Autodesk Inventor part; units mm, degrees
(part 2 of 6)
sketch "S03_340p2" plane through (0, 0, 0) normal (0, 0, 1) x (1, 0, 0)
  spline S0 degree 4 poles (238.0768, -5.4859) (238.0262, -5.474) (237.779, -5.4146) (237.364, -5.3165) (236.6634, -5.1506) (235.9264, -4.9756) (235.0209, -4.7632) (233.9546, -4.5121) (232.7252, -4.2255) (231.3359, -3.902) (229.7872, -3.5447) (228.0804, -3.1524) (226.2178, -2.7277) (224.2001, -2.2712) (222.0305, -1.7836) (219.7094, -1.2675) (217.2402, -0.7231) (214.625, -0.1526) (211.8658, 0.4439) (208.9653, 1.0631) (205.9266, 1.7045) (202.7523, 2.3663) (199.4449, 3.0472) (196.0087, 3.7454) (192.4456, 4.4591) (188.7604, 5.1862) (184.955, 5.9264) (181.0347, 6.6766) (177.0015, 7.4365) (172.8611, 8.2025) (168.6158, 8.9751) (164.2708, 9.7507) (159.8297, 10.529) (155.2973, 11.3074) (150.6772, 12.0849) (145.9752, 12.8596) (141.1941, 13.6294) (136.34, 14.3935) (131.4172, 15.1492) (126.4302, 15.8959) (121.3842, 16.6311) (116.2838, 17.3537) (111.1345, 18.0622) (105.9413, 18.7549) (100.7087, 19.4294) (95.443, 20.0851) (90.1479, 20.7208) (84.8303, 21.3331) (79.494, 21.9228) (74.1456, 22.4868) (68.7891, 23.0248) (63.4312, 23.5346) (58.0761, 24.0141) (52.7299, 24.4647) (47.3975, 24.8819) (42.08, 25.2672) (36.7914, 25.6169) (31.5078, 25.9337) (26.2453, 26.1996) (21.0236, 26.419) (15.8442, 26.589) (10.716, 26.7093) (5.6442, 26.7813) (0.6348, 26.8019) (-4.3081, 26.7748) (-9.1776, 26.6965) (-13.9701, 26.5701) (-18.6795, 26.3941) (-23.3014, 26.171) (-27.8303, 25.8995) (-32.2623, 25.5822) (-36.5918, 25.2189) (-40.8146, 24.8118) (-44.9265, 24.3608) (-48.9229, 23.8689) (-52.7993, 23.3366) (-56.5528, 22.7661) (-60.1783, 22.1582) (-63.673, 21.5164) (-67.0326, 20.8409) (-70.2544, 20.1338) (-73.3348, 19.3988) (-76.2708, 18.6358) (-79.0595, 17.8478) (-81.6988, 17.0376) (-84.1852, 16.2058) (-86.5171, 15.3554) (-88.6923, 14.4885) (-90.7089, 13.6063) (-92.5646, 12.7109) (-94.2592, 11.8045) (-95.7904, 10.8887) (-97.157, 9.9637) (-98.3599, 9.0328) (-99.3959, 8.0942) (-100.2663, 7.1501) (-100.9698, 6.2002) (-101.5046, 5.2436) (-101.867, 4.2806) (-102.0565, 3.315) (-102.0685, 2.3484) (-101.9089, 1.395) (-101.5753, 0.4697) (-101.0719, -0.4267) (-100.4022, -1.2915) (-99.569, -2.1257) (-98.5748, -2.9295) (-97.4206, -3.7051) (-96.1081, -4.4524) (-94.638, -5.1717) (-93.0118, -5.863) (-91.2313, -6.5259) (-89.2977, -7.1607) (-87.2135, -7.7667) (-84.9804, -8.3444) (-82.6012, -8.8925) (-80.0775, -9.4126) (-77.4128, -9.9023) (-74.609, -10.3636) (-71.6695, -10.7959) (-68.5965, -11.1986) (-65.3939, -11.5716) (-62.0641, -11.9176) (-58.6109, -12.2331) (-55.0375, -12.5221) (-51.3466, -12.7824) (-47.5428, -13.0161) (-43.6291, -13.2239) (-39.6094, -13.4046) (-35.4871, -13.5622) (-31.2664, -13.6937) (-26.9512, -13.8041) (-22.5454, -13.891) (-18.0526, -13.9576) (-13.4782, -14.005) (-8.8246, -14.0327) (-4.0979, -14.0442) (0.6989, -14.0393) (5.5607, -14.0194) (10.4834, -13.9869) (15.4623, -13.9431) (20.4929, -13.8877) (25.5736, -13.8249) (30.6965, -13.752) (35.87, -13.6774) (41.1014, -13.5853) (46.3548, -13.48) (51.6364, -13.3596) (56.934, -13.2271) (62.2443, -13.0833) (67.5615, -12.9292) (72.8799, -12.7653) (78.1948, -12.5938) (83.501, -12.4137) (88.7934, -12.2286) (94.0665, -12.0366) (99.3153, -11.8411) (104.5345, -11.6413) (109.7195, -11.4375) (114.8643, -11.2326) (119.9644, -11.0252) (125.0148, -10.816) (130.0105, -10.6074) (134.9458, -10.3977) (139.8171, -10.189) (144.6184, -9.9809) (149.3454, -9.7738) (153.9932, -9.5683) (158.5579, -9.365) (163.0336, -9.1642) (167.4168, -8.9655) (171.7029, -8.7695) (175.8874, -8.5777) (179.9659, -8.3878) (183.9349, -8.2029) (187.7897, -8.0209) (191.5269, -7.8443) (195.1424, -7.6707) (198.6328, -7.5029) (201.994, -7.3394) (205.2234, -7.1814) (208.3166, -7.0282) (211.2715, -6.8818) (214.0843, -6.7401) (216.7525, -6.6055) (219.2732, -6.4775) (221.6439, -6.3552) (223.8618, -6.2408) (225.9253, -6.1339) (227.8314, -6.0336) (229.5784, -5.9419) (231.1648, -5.8574) (232.5882, -5.7821) (233.848, -5.7143) (234.9418, -5.6556) (235.87, -5.6058) (236.6266, -5.5642) (237.3454, -5.5262) (237.7711, -5.5022) (238.0248, -5.4886) (238.0768, -5.4859) knots 0 0 0 0 0 0.003306 0.005253 0.00752 0.010062 0.01285 0.015861 0.019079 0.022488 0.026078 0.029837 0.033757 0.037828 0.042045 0.046398 0.050884 0.055494 0.060224 0.065069 0.070023 0.075082 0.080241 0.085495 0.090841 0.096274 0.101791 0.107386 0.113057 0.118799 0.124609 0.130484 0.136419 0.142412 0.148458 0.154554 0.160697 0.166884 0.17311 0.179374 0.185671 0.191998 0.198352 0.20473 0.211128 0.217543 0.223972 0.230412 0.23686 0.243312 0.249765 0.256217 0.262663 0.2691 0.275526 0.281941 0.288345 0.294734 0.301105 0.307451 0.313767 0.320049 0.326294 0.332498 0.338659 0.344773 0.350837 0.356848 0.362801 0.368695 0.374525 0.380288 0.38598 0.391599 0.39714 0.4026 0.407976 0.413263 0.418458 0.423557 0.428556 0.433452 0.438241 0.442917 0.447478 0.451919 0.456236 0.460425 0.464482 0.468403 0.472185 0.475825 0.479322 0.482675 0.485889 0.48897 0.49193 0.494788 0.497572 0.50031 0.503032 0.505769 0.508552 0.511409 0.514365 0.517441 0.520647 0.523991 0.527474 0.531098 0.534861 0.538758 0.542789 0.546947 0.551231 0.555634 0.560154 0.564786 0.569527 0.574371 0.579315 0.584356 0.58949 0.594712 0.60002 0.605409 0.610877 0.61642 0.622034 0.627716 0.633463 0.639271 0.645138 0.651061 0.657035 0.663059 0.669128 0.675241 0.681393 0.687582 0.693804 0.700057 0.706341 0.712655 0.718998 0.725365 0.731751 0.738149 0.744556 0.750969 0.757385 0.7638 0.770211 0.776616 0.783011 0.789393 0.795759 0.802106 0.808429 0.814727 0.820996 0.827232 0.833433 0.839595 0.845714 0.851788 0.857813 0.863785 0.869702 0.875558 0.881352 0.887078 0.892735 0.898316 0.90382 0.909242 0.914577 0.919822 0.924972 0.930023 0.93497 0.939808 0.944533 0.949139 0.95362 0.95797 0.962183 0.966252 0.970169 0.973927 0.977515 0.980924 0.984141 0.987151 0.989939 0.99248 0.994747 0.996694 1 1 1 1 1
  circle A0 centre (0, 0) radius 5.15
  line L0 (-36.89, 3.1) -> (-26.69, 3.1)
  line L1 (-26.69, 3.1) -> (-26.69, -1.1)
  line L2 (-26.69, -1.1) -> (-36.89, -1.1)
  line L3 (-36.89, -1.1) -> (-36.89, 3.1)
  line L4 (-36.89, 3.1) -> (-26.69, -1.1) construction
  line L5 (-26.69, 3.1) -> (-36.89, -1.1) construction
  line L6 (-73.14, 4.1) -> (-62.94, 4.1)
  line L7 (-62.94, 4.1) -> (-62.94, -0.1)
  line L8 (-62.94, -0.1) -> (-73.14, -0.1)
  line L9 (-73.14, -0.1) -> (-73.14, 4.1)
  line L10 (-73.14, 4.1) -> (-62.94, -0.1) construction
  line L11 (-62.94, 4.1) -> (-73.14, -0.1) construction
  line L12 (55.1, 4.1) -> (44.9, 4.1)
  line L13 (44.9, 4.1) -> (44.9, -0.1)
  line L14 (44.9, -0.1) -> (55.1, -0.1)
  line L15 (55.1, -0.1) -> (55.1, 4.1)
  line L16 (55.1, 4.1) -> (44.9, -0.1) construction
  line L17 (44.9, 4.1) -> (55.1, -0.1) construction
  line L18 (114.9, -0.1) -> (125.1, -0.1)
  line L19 (125.1, -0.1) -> (125.1, 4.1)
  line L20 (125.1, 4.1) -> (114.9, 4.1)
  line L21 (114.9, 4.1) -> (114.9, -0.1)
  line L22 (114.9, -0.1) -> (125.1, 4.1) construction
  line L23 (125.1, -0.1) -> (114.9, 4.1) construction
  point P0 (237.7462, -5.4071)
  point P1 (237.3329, -5.3091)
  point P2 (236.7552, -5.1723)
  point P3 (236.0133, -4.9966)
  point P4 (235.108, -4.7835)
  point P5 (234.0398, -4.5326)
  point P6 (232.8098, -4.2453)
  point P7 (231.4193, -3.922)
  point P8 (229.8697, -3.564)
  point P9 (228.162, -3.1718)
  point P10 (226.2982, -2.7467)
  point P11 (224.2795, -2.2898)
  point P12 (222.1085, -1.8021)
  point P13 (219.7863, -1.2855)
  point P14 (217.3158, -0.7409)
  point P15 (214.6992, -0.1699)
  point P16 (211.9385, 0.4267)
  point P17 (209.0365, 1.0465)
  point P18 (205.9962, 1.6882)
  point P19 (202.8202, 2.3505)
  point P20 (199.5113, 3.0317)
  point P21 (196.0731, 3.7303)
  point P22 (192.5083, 4.4444)
  point P23 (188.821, 5.1721)
  point P24 (185.0139, 5.9125)
  point P25 (181.0913, 6.6634)
  point P26 (177.0563, 7.4234)
  point P27 (172.9136, 8.1902)
  point P28 (168.6662, 8.9629)
  point P29 (164.3189, 9.7392)
  point P30 (159.8756, 10.5178)
  point P31 (155.3408, 11.2967)
  point P32 (150.7185, 12.0746)
  point P33 (146.0138, 12.8496)
  point P34 (141.2304, 13.62)
  point P35 (136.3737, 14.3843)
  point P36 (131.4484, 15.1406)
  point P37 (126.459, 15.8875)
  point P38 (121.4103, 16.6231)
  point P39 (116.3073, 17.3461)
  point P40 (111.1553, 18.0549)
  point P41 (105.9594, 18.7476)
  point P42 (100.7243, 19.4226)
  point P43 (95.4557, 20.0786)
  point P44 (90.1581, 20.7142)
  point P45 (84.8375, 21.3271)
  point P46 (79.4986, 21.9167)
  point P47 (74.1473, 22.481)
  point P48 (68.7882, 23.019)
  point P49 (63.4275, 23.5287)
  point P50 (58.0698, 24.0088)
  point P51 (52.7209, 24.4587)
  point P52 (47.3859, 24.8763)
  point P53 (42.0706, 25.2608)
  point P54 (36.78, 25.6108)
  point P55 (31.4944, 25.9241)
  point P56 (26.2263, 26.1912)
  point P57 (20.9987, 26.41)
  point P58 (15.8166, 26.5797)
  point P59 (10.6858, 26.7)
  point P60 (5.6116, 26.771)
  point P61 (0.5997, 26.7919)
  point P62 (-4.3454, 26.7636)
  point P63 (-9.2175, 26.6853)
  point P64 (-14.012, 26.5579)
  point P65 (-18.7237, 26.3816)
  point P66 (-23.3476, 26.1574)
  point P67 (-27.8787, 25.8855)
  point P68 (-32.3125, 25.567)
  point P69 (-36.644, 25.203)
  point P70 (-40.8685, 24.7947)
  point P71 (-44.9822, 24.343)
  point P72 (-48.98, 23.8498)
  point P73 (-52.858, 23.3164)
  point P74 (-56.6127, 22.7445)
  point P75 (-60.2396, 22.1356)
  point P76 (-63.7352, 21.492)
  point P77 (-67.0959, 20.815)
  point P78 (-70.3184, 20.1066)
  point P79 (-73.3994, 19.3694)
  point P80 (-76.3357, 18.6047)
  point P81 (-79.1245, 17.8148)
  point P82 (-81.7635, 17.0021)
  point P83 (-84.2495, 16.1682)
  point P84 (-86.5804, 15.3153)
  point P85 (-88.7541, 14.4456)
  point P86 (-90.7686, 13.5607)
  point P87 (-92.6218, 12.6625)
  point P88 (-94.3125, 11.753)
  point P89 (-95.8388, 10.834)
  point P90 (-97.1996, 9.9068)
  point P91 (-98.394, 8.9733)
  point P92 (-99.4206, 8.0343)
  point P93 (-100.2791, 7.0914)
  point P94 (-100.9688, 6.146)
  point P95 (-101.4892, 5.1984)
  point P96 (-101.8398, 4.2495)
  point P97 (-102.0213, 3.3002)
  point P98 (-102.0329, 2.3511)
  point P99 (-101.8765, 1.4147)
  point P100 (-101.5531, 0.5042)
  point P101 (-101.0638, -0.3803)
  point P102 (-100.4091, -1.2386)
  point P103 (-99.5898, -2.0705)
  point P104 (-98.6072, -2.8751)
  point P105 (-97.4623, -3.6528)
  point P106 (-96.1569, -4.4033)
  point P107 (-94.6923, -5.1261)
  point P108 (-93.0701, -5.821)
  point P109 (-91.2925, -6.4874)
  point P110 (-89.3611, -7.1253)
  point P111 (-87.2782, -7.7345)
  point P112 (-85.046, -8.3147)
  point P113 (-82.6672, -8.8657)
  point P114 (-80.1437, -9.3876)
  point P115 (-77.4787, -9.8799)
  point P116 (-74.6744, -10.343)
  point P117 (-71.7341, -10.7769)
  point P118 (-68.6604, -11.1812)
  point P119 (-65.4567, -11.5561)
  point P120 (-62.1258, -11.9027)
  point P121 (-58.6713, -12.2202)
  point P122 (-55.0964, -12.5098)
  point P123 (-51.4042, -12.7715)
  point P124 (-47.5987, -13.0062)
  point P125 (-43.6833, -13.2145)
  point P126 (-39.6619, -13.3967)
  point P127 (-35.5378, -13.5543)
  point P128 (-31.3152, -13.6873)
  point P129 (-26.9981, -13.7977)
  point P130 (-22.5903, -13.8857)
  point P131 (-18.0955, -13.9528)
  point P132 (-13.5187, -14.0004)
  point P133 (-8.8632, -14.0291)
  point P134 (-4.1341, -14.0407)
  point P135 (0.6648, -14.0363)
  point P136 (5.529, -14.017)
  point P137 (10.4541, -13.9849)
  point P138 (15.4352, -13.9411)
  point P139 (20.468, -13.8866)
  point P140 (25.548, -13.8233)
  point P141 (30.6703, -13.7521)
  point P142 (35.8472, -13.6743)
  point P143 (41.0816, -13.583)
  point P144 (46.3429, -13.4772)
  point P145 (51.627, -13.3574)
  point P146 (56.9277, -13.225)
  point P147 (62.2405, -13.0813)
  point P148 (67.5604, -12.9272)
  point P149 (72.8816, -12.7636)
  point P150 (78.1992, -12.5918)
  point P151 (83.5081, -12.4123)
  point P152 (88.8032, -12.2267)
  point P153 (94.0791, -12.0352)
  point P154 (99.3305, -11.8394)
  point P155 (104.5524, -11.6395)
  point P156 (109.7401, -11.4361)
  point P157 (114.8876, -11.2308)
  point P158 (119.9903, -11.0234)
  point P159 (125.0433, -10.8145)
  point P160 (130.0416, -10.6054)
  point P161 (134.9796, -10.3959)
  point P162 (139.8533, -10.1869)
  point P163 (144.6572, -9.9788)
  point P164 (149.3865, -9.7716)
  point P165 (154.0369, -9.5661)
  point P166 (158.6039, -9.3626)
  point P167 (163.082, -9.1616)
  point P168 (167.4674, -8.9629)
  point P169 (171.7559, -8.767)
  point P170 (175.9425, -8.5746)
  point P171 (180.0232, -8.3851)
  point P172 (183.9942, -8.1996)
  point P173 (187.8512, -8.018)
  point P174 (191.5903, -7.8407)
  point P175 (195.2078, -7.6675)
  point P176 (198.7, -7.4992)
  point P177 (202.0631, -7.3358)
  point P178 (205.2941, -7.1775)
  point P179 (208.3891, -7.0246)
  point P180 (211.3456, -6.8776)
  point P181 (214.16, -6.7363)
  point P182 (216.8296, -6.6014)
  point P183 (219.3517, -6.4731)
  point P184 (221.7236, -6.3511)
  point P185 (223.9429, -6.2365)
  point P186 (226.0075, -6.1293)
  point P187 (227.9148, -6.0293)
  point P188 (229.6629, -5.9372)
  point P189 (231.2503, -5.853)
  point P190 (232.6748, -5.7772)
  point P191 (233.9354, -5.7096)
  point P192 (235.0308, -5.6508)
  point P193 (235.9593, -5.6008)
  point P194 (236.7208, -5.5594)
  point P195 (237.3136, -5.5275)
  point P196 (237.7375, -5.5042)
  point P197 (237.992, -5.4904)
  point P198 (-31.79, 1)
  point P199 (-68.04, 2)
  dimension "d4" = 10.3
  dimension "d5" = 102.06
  dimension "d51" = 10.2
  dimension "d52" = 4.2
  dimension "d54" = 10.2
  dimension "d55" = 4.2
  dimension "d130" = -31.79
  dimension "d131" = 1
  dimension "d132" = -68.04
  dimension "d133" = 2
  dimension "d203" = 10.2
  dimension "d204" = 4.2
  dimension "d205" = 50
  dimension "d206" = 2
  dimension "d207" = 10.2
  dimension "d208" = 4.2
  dimension "d209" = 120
  dimension "d210" = 2
  constraints: 48 end point, 8 midpoint, 8 parallel, 4 horizontal, 4 perpendicular, 1 centre point, 201 other
  measures "d4" diameter of A0
  measures "d5" distance of A0.centre point (-102.033, 2.351)
  measures "d51" distance of L1.end L2.end
  measures "d52" distance of L0.end L1.end
  measures "d54" distance of L7.end L8.end
  measures "d55" distance of L6.end L7.end
  measures "d130" horizontal distance of point (0, 0) point (-31.79, 1)
  measures "d131" vertical distance of point (0, 0) point (-31.79, 1)
  measures "d132" horizontal distance of point (0, 0) point (-68.04, 2)
  measures "d133" vertical distance of point (0, 0) point (-68.04, 2)
  measures "d203" distance of L14.end L13.end
  measures "d204" distance of L13.end L12.end
  measures "d205" horizontal distance of point (0, 0) point (50, 2)
  measures "d206" vertical distance of point (0, 0) point (50, 2)
  measures "d207" distance of L20.end L19.end
  measures "d208" distance of L19.end L18.end
  measures "d209" horizontal distance of point (120, 2) point (0, 0)
  measures "d210" vertical distance of point (0, 0) point (120, 2)
sketch "S04_341p5" plane through (0, 0, 0) normal (0, 0, 1) x (1, 0, 0)
  spline S0 degree 4 poles (238.894, -8.6346) (238.8434, -8.6221) (238.596, -8.5592) (238.1807, -8.4553) (237.4798, -8.2795) (236.7423, -8.0942) (235.8362, -7.8691) (234.7692, -7.603) (233.539, -7.2992) (232.1488, -6.9562) (230.599, -6.5773) (228.891, -6.1611) (227.0269, -5.7103) (225.0077, -5.2256) (222.8364, -4.7076) (220.5134, -4.1592) (218.0422, -3.5803) (215.4246, -2.9733) (212.663, -2.3383) (209.7598, -1.6786) (206.7181, -0.9949) (203.5407, -0.289) (200.2299, 0.438) (196.7901, 1.1839) (193.223, 1.9471) (189.5336, 2.7253) (185.7237, 3.5183) (181.7986, 4.3229) (177.7604, 5.1385) (173.6146, 5.9618) (169.3635, 6.793) (165.0125, 7.6287) (160.565, 8.4682) (156.026, 9.3091) (151.3988, 10.1502) (146.6894, 10.9896) (141.9006, 11.8251) (137.0383, 12.6558) (132.1071, 13.4791) (127.1113, 14.294) (122.0562, 15.0983) (116.9462, 15.8906) (111.7869, 16.6694) (106.5835, 17.4329) (101.3402, 18.1787) (96.0635, 18.906) (90.7569, 19.6137) (85.4274, 20.2981) (80.079, 20.9602) (74.718, 21.5965) (69.3485, 22.2069) (63.9774, 22.7891) (58.6086, 23.3407) (53.2483, 23.8632) (47.9015, 24.3521) (42.5692, 24.8087) (37.2654, 25.2291) (31.9662, 25.6166) (26.6876, 25.9526) (21.4493, 26.2414) (16.2527, 26.4802) (11.107, 26.6682) (6.0172, 26.8071) (0.9893, 26.8936) (-3.9724, 26.9314) (-8.8611, 26.9168) (-13.6732, 26.8529) (-18.4024, 26.7382) (-23.0446, 26.575) (-27.594, 26.362) (-32.0467, 26.1016) (-36.3971, 25.7939) (-40.641, 25.4408) (-44.7743, 25.0421) (-48.792, 24.6009) (-52.6899, 24.1175) (-56.4649, 23.5942) (-60.1119, 23.0317) (-63.6281, 22.4334) (-67.0092, 21.7996) (-70.2523, 21.1321) (-73.3539, 20.4348) (-76.3109, 19.7076) (-79.1203, 18.9533) (-81.7801, 18.1747) (-84.2867, 17.3725) (-86.6385, 16.5496) (-88.8332, 15.708) (-90.8689, 14.849) (-92.7434, 13.9747) (-94.4562, 13.0872) (-96.0051, 12.188) (-97.389, 11.2775) (-98.6086, 10.3589) (-99.6608, 9.4305) (-100.5469, 8.4942) (-101.2655, 7.5501) (-101.8149, 6.5969) (-102.1912, 5.6351) (-102.3942, 4.6684) (-102.4189, 3.6983) (-102.2712, 2.7392) (-101.9486, 1.8061) (-101.455, 0.8998) (-100.7942, 0.0229) (-99.9689, -0.8254) (-98.9815, -1.6453) (-97.8332, -2.4388) (-96.5256, -3.2062) (-95.0595, -3.9475) (-93.4363, -4.6627) (-91.6578, -5.3515) (-89.7253, -6.0141) (-87.6413, -6.6498) (-85.4074, -7.259) (-83.0265, -7.8404) (-80.5003, -8.3956) (-77.8321, -8.9221) (-75.0238, -9.422) (-72.079, -9.8945) (-68.9999, -10.3391) (-65.7902, -10.7556) (-62.4525, -11.1466) (-58.9906, -11.5087) (-55.4076, -11.8457) (-51.7064, -12.1555) (-47.8914, -12.4401) (-43.9658, -12.7) (-39.9335, -12.9342) (-35.7979, -13.1466) (-31.5631, -13.334) (-27.2332, -13.5015) (-22.8122, -13.6466) (-18.3035, -13.7725) (-13.7125, -13.8802) (-9.0419, -13.9692) (-4.2977, -14.0428) (0.517, -14.1009) (5.3973, -14.1449) (10.3388, -14.1769) (15.3368, -14.1983) (20.387, -14.2089) (25.4875, -14.2125) (30.6305, -14.2067) (35.8243, -14.1998) (41.0764, -14.1761) (46.3508, -14.1394) (51.6538, -14.088) (56.9729, -14.0246) (62.3049, -13.95) (67.644, -13.8653) (72.9844, -13.7706) (78.3214, -13.6683) (83.6498, -13.5573) (88.9644, -13.441) (94.2597, -13.3175) (99.5307, -13.1903) (104.772, -13.0584) (109.9791, -12.9219) (115.1458, -12.7838) (120.2677, -12.6427) (125.3396, -12.4991) (130.3568, -12.3554) (135.3133, -12.2096) (140.2055, -12.0642) (145.0275, -11.9185) (149.7748, -11.7727) (154.4427, -11.6274) (159.0271, -11.4834) (163.5221, -11.3407) (167.9243, -11.1988) (172.2291, -11.0584) (176.4316, -10.9208) (180.5279, -10.7839) (184.5141, -10.6504) (188.3858, -10.5184) (192.1392, -10.3902) (195.7705, -10.2635) (199.2762, -10.1409) (202.6521, -10.0209) (205.8956, -9.9047) (209.0024, -9.7916) (211.9703, -9.6836) (214.7954, -9.5783) (217.4754, -9.4782) (220.0072, -9.3828) (222.3883, -9.2913) (224.616, -9.2056) (226.6886, -9.1253) (228.6031, -9.0498) (230.3579, -8.9807) (231.9513, -8.9167) (233.381, -8.8598) (234.6464, -8.8083) (235.7451, -8.7638) (236.6773, -8.726) (237.4373, -8.6942) (238.1594, -8.6654) (238.587, -8.647) (238.8418, -8.6366) (238.894, -8.6346) knots 0 0 0 0 0 0.003306 0.005253 0.00752 0.010062 0.01285 0.015861 0.019079 0.022488 0.026078 0.029837 0.033757 0.037828 0.042045 0.046398 0.050884 0.055494 0.060224 0.065069 0.070023 0.075082 0.080241 0.085495 0.090841 0.096274 0.101791 0.107386 0.113057 0.118799 0.124609 0.130484 0.136419 0.142412 0.148458 0.154554 0.160697 0.166884 0.17311 0.179374 0.185671 0.191998 0.198352 0.20473 0.211128 0.217543 0.223972 0.230412 0.23686 0.243312 0.249765 0.256217 0.262663 0.2691 0.275526 0.281941 0.288345 0.294734 0.301105 0.307451 0.313767 0.320049 0.326294 0.332498 0.338659 0.344773 0.350837 0.356848 0.362801 0.368695 0.374525 0.380288 0.38598 0.391599 0.39714 0.4026 0.407976 0.413263 0.418458 0.423557 0.428556 0.433452 0.438241 0.442917 0.447478 0.451919 0.456236 0.460425 0.464482 0.468403 0.472185 0.475825 0.479322 0.482675 0.485889 0.48897 0.49193 0.494788 0.497572 0.50031 0.503032 0.505769 0.508552 0.511409 0.514365 0.517441 0.520647 0.523991 0.527474 0.531098 0.534861 0.538758 0.542789 0.546947 0.551231 0.555634 0.560154 0.564786 0.569527 0.574371 0.579315 0.584356 0.58949 0.594712 0.60002 0.605409 0.610877 0.61642 0.622034 0.627716 0.633463 0.639271 0.645138 0.651061 0.657035 0.663059 0.669128 0.675241 0.681393 0.687582 0.693804 0.700057 0.706341 0.712655 0.718998 0.725365 0.731751 0.738149 0.744556 0.750969 0.757385 0.7638 0.770211 0.776616 0.783011 0.789393 0.795759 0.802106 0.808429 0.814727 0.820996 0.827232 0.833433 0.839595 0.845714 0.851788 0.857813 0.863785 0.869702 0.875558 0.881352 0.887078 0.892735 0.898316 0.90382 0.909242 0.914577 0.919822 0.924972 0.930023 0.93497 0.939808 0.944533 0.949139 0.95362 0.95797 0.962183 0.966252 0.970169 0.973927 0.977515 0.980924 0.984141 0.987151 0.989939 0.99248 0.994747 0.996694 1 1 1 1 1
  circle A0 centre (0, 0) radius 5.15
  line L0 (-62.94, -0.1) -> (-73.14, -0.1)
  line L1 (-73.14, -0.1) -> (-73.14, 4.1)
  line L2 (-73.14, 4.1) -> (-62.94, 4.1)
  line L3 (-62.94, 4.1) -> (-62.94, -0.1)
  line L4 (-62.94, -0.1) -> (-73.14, 4.1) construction
  line L5 (-73.14, -0.1) -> (-62.94, 4.1) construction
  line L6 (-39.25, 0.9) -> (-29.05, 0.9)
  line L7 (-29.05, 0.9) -> (-29.05, 5.1)
  line L8 (-29.05, 5.1) -> (-39.25, 5.1)
  line L9 (-39.25, 5.1) -> (-39.25, 0.9)
  line L10 (-39.25, 0.9) -> (-29.05, 5.1) construction
  line L11 (-29.05, 0.9) -> (-39.25, 5.1) construction
  line L12 (125.1, 4.1) -> (114.9, 4.1)
  line L13 (114.9, 4.1) -> (114.9, -0.1)
  line L14 (114.9, -0.1) -> (125.1, -0.1)
  line L15 (125.1, -0.1) -> (125.1, 4.1)
  line L16 (125.1, 4.1) -> (114.9, -0.1) construction
  line L17 (114.9, 4.1) -> (125.1, -0.1) construction
  line L18 (65.1, 4.1) -> (54.9, 4.1)
  line L19 (54.9, 4.1) -> (54.9, -0.1)
  line L20 (54.9, -0.1) -> (65.1, -0.1)
  line L21 (65.1, -0.1) -> (65.1, 4.1)
  line L22 (65.1, 4.1) -> (54.9, -0.1) construction
  line L23 (54.9, 4.1) -> (65.1, -0.1) construction
  point P0 (238.5632, -8.5512)
  point P1 (238.1497, -8.4474)
  point P2 (237.5716, -8.3025)
  point P3 (236.8293, -8.1164)
  point P4 (235.9233, -7.8906)
  point P5 (234.8544, -7.6247)
  point P6 (233.6236, -7.3202)
  point P7 (232.2322, -6.9774)
  point P8 (230.6815, -6.5977)
  point P9 (228.9726, -6.1816)
  point P10 (227.1074, -5.7304)
  point P11 (225.0872, -5.2453)
  point P12 (222.9145, -4.7273)
  point P13 (220.5904, -4.1782)
  point P14 (218.1178, -3.5991)
  point P15 (215.4989, -2.9916)
  point P16 (212.7358, -2.3565)
  point P17 (209.8311, -1.6963)
  point P18 (206.7878, -1.0122)
  point P19 (203.6087, -0.3057)
  point P20 (200.2963, 0.4216)
  point P21 (196.8545, 1.1679)
  point P22 (193.2858, 1.9315)
  point P23 (189.5943, 2.7104)
  point P24 (185.7827, 3.5036)
  point P25 (181.8553, 4.3088)
  point P26 (177.8152, 5.1246)
  point P27 (173.6671, 5.9488)
  point P28 (169.414, 6.7802)
  point P29 (165.0606, 7.6165)
  point P30 (160.611, 8.4563)
  point P31 (156.0695, 9.2978)
  point P32 (151.4402, 10.1393)
  point P33 (146.7281, 10.9791)
  point P34 (141.9369, 11.8152)
  point P35 (137.0721, 12.6461)
  point P36 (132.1384, 13.4699)
  point P37 (127.1401, 14.2852)
  point P38 (122.0823, 15.0899)
  point P39 (116.9697, 15.8826)
  point P40 (111.8078, 16.6618)
  point P41 (106.6015, 17.4254)
  point P42 (101.3557, 18.1717)
  point P43 (96.0761, 18.8993)
  point P44 (90.767, 19.6069)
  point P45 (85.4346, 20.2921)
  point P46 (80.0836, 20.954)
  point P47 (74.7197, 21.5907)
  point P48 (69.3476, 22.2011)
  point P49 (63.9735, 22.7832)
  point P50 (58.6021, 23.3355)
  point P51 (53.2392, 23.8574)
  point P52 (47.8898, 24.3466)
  point P53 (42.5597, 24.8024)
  point P54 (37.2539, 25.2231)
  point P55 (31.9526, 25.6071)
  point P56 (26.6685, 25.9444)
  point P57 (21.4242, 26.2327)
  point P58 (16.225, 26.4712)
  point P59 (11.0765, 26.6593)
  point P60 (5.9844, 26.7972)
  point P61 (0.9539, 26.8841)
  point P62 (-4.01, 26.9206)
  point P63 (-8.9013, 26.9061)
  point P64 (-13.7154, 26.8412)
  point P65 (-18.4469, 26.7262)
  point P66 (-23.0911, 26.5619)
  point P67 (-27.6427, 26.3485)
  point P68 (-32.0973, 26.0871)
  point P69 (-36.4497, 25.7787)
  point P70 (-40.6954, 25.4243)
  point P71 (-44.8303, 25.025)
  point P72 (-48.8496, 24.5825)
  point P73 (-52.7491, 24.0981)
  point P74 (-56.5253, 23.5733)
  point P75 (-60.1737, 23.0098)
  point P76 (-63.6909, 22.4097)
  point P77 (-67.073, 21.7744)
  point P78 (-70.3169, 21.1056)
  point P79 (-73.4191, 20.4062)
  point P80 (-76.3764, 19.6772)
  point P81 (-79.186, 18.921)
  point P82 (-81.8455, 18.14)
  point P83 (-84.3517, 17.3356)
  point P84 (-86.7025, 16.5102)
  point P85 (-88.8958, 15.6658)
  point P86 (-90.9295, 14.804)
  point P87 (-92.8014, 13.9268)
  point P88 (-94.5104, 13.0362)
  point P89 (-96.0544, 12.1338)
  point P90 (-97.4325, 11.221)
  point P91 (-98.6437, 10.2997)
  point P92 (-99.6864, 9.3707)
  point P93 (-100.5605, 8.4355)
  point P94 (-101.2652, 7.4956)
  point P95 (-101.8, 6.5513)
  point P96 (-102.1643, 5.6035)
  point P97 (-102.359, 4.6531)
  point P98 (-102.3831, 3.7005)
  point P99 (-102.2385, 2.7586)
  point P100 (-101.9258, 1.8404)
  point P101 (-101.4463, 0.9462)
  point P102 (-100.8004, 0.0761)
  point P103 (-99.989, -0.7696)
  point P104 (-99.0133, -1.5902)
  point P105 (-97.8744, -2.3859)
  point P106 (-96.5739, -3.1563)
  point P107 (-95.1133, -3.9011)
  point P108 (-93.4943, -4.6198)
  point P109 (-91.7187, -5.3121)
  point P110 (-89.7885, -5.9778)
  point P111 (-87.7059, -6.6166)
  point P112 (-85.473, -7.2283)
  point P113 (-83.0925, -7.8126)
  point P114 (-80.5664, -8.3696)
  point P115 (-77.8979, -8.8987)
  point P116 (-75.0893, -9.4004)
  point P117 (-72.1437, -9.8746)
  point P118 (-69.0638, -10.3208)
  point P119 (-65.8531, -10.7392)
  point P120 (-62.5142, -11.1309)
  point P121 (-59.051, -11.4949)
  point P122 (-55.4666, -11.8326)
  point P123 (-51.764, -12.1438)
  point P124 (-47.9474, -12.4294)
  point P125 (-44.0201, -12.6899)
  point P126 (-39.9861, -12.9256)
  point P127 (-35.8487, -13.138)
  point P128 (-31.612, -13.327)
  point P129 (-27.2802, -13.4945)
  point P130 (-22.8571, -13.6407)
  point P131 (-18.3465, -13.7672)
  point P132 (-13.7532, -13.8751)
  point P133 (-9.0806, -13.965)
  point P134 (-4.334, -14.0389)
  point P135 (0.4828, -14.0975)
  point P136 (5.3655, -14.142)
  point P137 (10.3094, -14.1745)
  point P138 (15.3097, -14.196)
  point P139 (20.362, -14.2074)
  point P140 (25.4618, -14.2106)
  point P141 (30.6042, -14.2065)
  point P142 (35.8014, -14.1964)
  point P143 (41.0566, -14.1735)
  point P144 (46.3389, -14.1365)
  point P145 (51.6443, -14.0856)
  point P146 (56.9665, -14.0224)
  point P147 (62.3011, -13.948)
  point P148 (67.6429, -13.8632)
  point P149 (72.9861, -13.769)
  point P150 (78.3258, -13.6664)
  point P151 (83.6569, -13.5559)
  point P152 (88.9743, -13.4392)
  point P153 (94.2723, -13.3163)
  point P154 (99.546, -13.1888)
  point P155 (104.79, -13.0568)
  point P156 (109.9997, -12.9208)
  point P157 (115.1692, -12.7823)
  point P158 (120.2937, -12.6412)
  point P159 (125.3683, -12.4979)
  point P160 (130.3879, -12.3537)
  point P161 (135.3472, -12.2083)
  point P162 (140.2418, -12.0626)
  point P163 (145.0664, -11.9168)
  point P164 (149.8161, -11.771)
  point P165 (154.4866, -11.6258)
  point P166 (159.0733, -11.4816)
  point P167 (163.5707, -11.3387)
  point P168 (167.9752, -11.1968)
  point P169 (172.2822, -11.0565)
  point P170 (176.487, -10.9184)
  point P171 (180.5854, -10.7819)
  point P172 (184.5737, -10.6479)
  point P173 (188.4475, -10.5162)
  point P174 (192.2029, -10.3875)
  point P175 (195.8362, -10.2611)
  point P176 (199.3437, -10.1381)
  point P177 (202.7215, -10.0182)
  point P178 (205.9666, -9.9018)
  point P179 (209.0752, -9.789)
  point P180 (212.0446, -9.6803)
  point P181 (214.8714, -9.5754)
  point P182 (217.5528, -9.4751)
  point P183 (220.086, -9.3794)
  point P184 (222.4684, -9.2882)
  point P185 (224.6974, -9.2023)
  point P186 (226.7712, -9.1218)
  point P187 (228.6869, -9.0465)
  point P188 (230.4428, -8.977)
  point P189 (232.0372, -8.9134)
  point P190 (233.468, -8.8561)
  point P191 (234.7342, -8.8048)
  point P192 (235.8345, -8.7601)
  point P193 (236.767, -8.7221)
  point P194 (237.5319, -8.6906)
  point P195 (238.1274, -8.6663)
  point P196 (238.5531, -8.6486)
  point P197 (238.8088, -8.638)
  point P198 (-68.04, 2)
  point P199 (-34.15, 3)
  dimension "d6" = 10.3
  dimension "d7" = 102.45
  dimension "d57" = 10.2
  dimension "d58" = 4.2
  dimension "d60" = 10.2
  dimension "d61" = 4.2
  dimension "d134" = -68.04
  dimension "d135" = 2
  dimension "d136" = 34.15
  dimension "d137" = 3
  dimension "d211" = 10.2
  dimension "d212" = 4.2
  dimension "d213" = 120
  dimension "d214" = 2
  dimension "d215" = 10.2
  dimension "d216" = 4.2
  dimension "d217" = 60
  dimension "d218" = 2
  constraints: 48 end point, 8 midpoint, 8 parallel, 4 horizontal, 4 perpendicular, 1 centre point, 201 other
  measures "d6" diameter of A0
  measures "d7" distance of A0.centre point (-102.383, 3.701)
  measures "d57" distance of L1.end L2.end
  measures "d58" distance of L0.end L1.end
  measures "d60" distance of L8.end L7.end
  measures "d61" distance of L7.end L6.end
  measures "d134" horizontal distance of point (0, 0) point (-68.04, 2)
  measures "d135" vertical distance of point (0, 0) point (-68.04, 2)
  measures "d136" horizontal distance of point (0, 0) point (-34.15, 3)
  measures "d137" vertical distance of point (0, 0) point (-34.15, 3)
  measures "d211" distance of L14.end L13.end
  measures "d212" distance of L13.end L12.end
  measures "d213" horizontal distance of point (0, 0) point (120, 2)
  measures "d214" vertical distance of point (0, 0) point (120, 2)
  measures "d215" distance of L20.end L19.end
  measures "d216" distance of L19.end L18.end
  measures "d217" horizontal distance of point (60, 2) point (0, 0)
  measures "d218" vertical distance of point (0, 0) point (60, 2)
sketch "S05_329p0" plane through (0, 0, 0) normal (0, 0, 1) x (1, 0, 0)
  spline S0 degree 4 poles (229.8922, -13.6984) (229.8438, -13.6852) (229.607, -13.619) (229.2093, -13.5096) (228.5381, -13.3245) (227.832, -13.1294) (226.9644, -12.8922) (225.9427, -12.6119) (224.7648, -12.2916) (223.4335, -11.9299) (221.9494, -11.53) (220.3137, -11.0907) (218.5286, -10.6145) (216.5947, -10.1022) (214.5151, -9.5544) (212.2901, -8.9738) (209.923, -8.3606) (207.4157, -7.717) (204.7702, -7.0433) (201.9889, -6.3425) (199.0747, -5.6154) (196.0303, -4.8639) (192.858, -4.0892) (189.5618, -3.2933) (186.1434, -2.4779) (182.6075, -1.6452) (178.956, -0.7956) (175.1937, 0.0677) (171.3227, 0.9443) (167.3483, 1.8306) (163.2727, 2.727) (159.1009, 3.6298) (154.8363, 4.5386) (150.4835, 5.4507) (146.0459, 6.3651) (141.529, 7.2797) (136.9356, 8.1922) (132.2713, 9.1018) (127.5404, 10.0059) (122.7471, 10.9033) (117.8965, 11.7919) (112.9928, 12.6701) (108.0413, 13.5364) (103.0469, 14.3889) (98.0136, 15.2254) (92.9479, 16.0448) (87.8529, 16.8459) (82.7353, 17.6252) (77.5989, 18.3833) (72.4499, 19.117) (67.2922, 19.8258) (62.1322, 20.5076) (56.9738, 21.1598) (51.8229, 21.7838) (46.6842, 22.3751) (41.5587, 22.935) (36.46, 23.4594) (31.3648, 23.952) (26.2884, 24.3946) (21.2497, 24.7907) (16.2501, 25.1378) (11.2984, 25.4348) (6.3993, 25.6833) (1.5588, 25.8799) (-3.2192, 26.0281) (-7.928, 26.1241) (-12.5641, 26.171) (-17.1216, 26.167) (-21.5963, 26.1144) (-25.9828, 26.0118) (-30.2771, 25.8613) (-34.4742, 25.6629) (-38.5696, 25.4185) (-42.5594, 25.1276) (-46.4389, 24.7932) (-50.204, 24.4154) (-53.8516, 23.9965) (-57.3769, 23.5369) (-60.7769, 23.0398) (-64.0476, 22.5056) (-67.1862, 21.9358) (-70.1892, 21.3341) (-73.0535, 20.7003) (-75.7764, 20.0371) (-78.3557, 19.3471) (-80.7879, 18.6309) (-83.0716, 17.8914) (-85.2043, 17.1302) (-87.1844, 16.3488) (-89.0094, 15.5489) (-90.679, 14.7327) (-92.1911, 13.9016) (-93.5445, 13.0558) (-94.7398, 12.1986) (-95.7742, 11.3281) (-96.6487, 10.4463) (-97.3621, 9.5532) (-97.9127, 8.6475) (-98.2968, 7.7296) (-98.5141, 6.8031) (-98.5597, 5.8694) (-98.4391, 4.9423) (-98.1494, 4.0363) (-97.6945, 3.1523) (-97.0777, 2.2929) (-96.3019, 1.4573) (-95.3694, 0.6454) (-94.2813, -0.1448) (-93.0392, -0.9133) (-91.6439, -1.6603) (-90.0966, -2.3858) (-88.3992, -3.0892) (-86.5529, -3.771) (-84.5601, -4.4301) (-82.4223, -5.0672) (-80.1423, -5.6808) (-77.7217, -6.2724) (-75.1637, -6.8397) (-72.4702, -7.3844) (-69.6446, -7.9058) (-66.689, -8.4034) (-63.6071, -8.8769) (-60.4012, -9.3287) (-57.0751, -9.7554) (-53.6318, -10.1607) (-50.074, -10.5424) (-46.4061, -10.9025) (-42.631, -11.2413) (-38.7527, -11.5577) (-34.7743, -11.8554) (-30.6999, -12.1314) (-26.5334, -12.3902) (-22.2786, -12.6296) (-17.939, -12.8524) (-13.5197, -13.0595) (-9.0233, -13.2505) (-4.4557, -13.4283) (0.1803, -13.5927) (4.8796, -13.745) (9.6382, -13.8872) (14.4515, -14.0204) (19.3153, -14.1443) (24.2277, -14.2628) (29.1811, -14.373) (34.1836, -14.4834) (39.2427, -14.5789) (44.3235, -14.6624) (49.4321, -14.7323) (54.5565, -14.7911) (59.6936, -14.8394) (64.8378, -14.8781) (69.9834, -14.9072) (75.126, -14.9289) (80.2605, -14.942) (85.3818, -14.9498) (90.4846, -14.9502) (95.5642, -14.9464) (100.6152, -14.9374) (105.6334, -14.9233) (110.6127, -14.9067) (115.549, -14.8862) (120.4372, -14.8621) (125.2726, -14.8367) (130.0496, -14.808) (134.7648, -14.7782) (139.4123, -14.7464) (143.9879, -14.713) (148.487, -14.6783) (152.9056, -14.6428) (157.2381, -14.6066) (161.4812, -14.5692) (165.6304, -14.5309) (169.6812, -14.4931) (173.6295, -14.4535) (177.4718, -14.4147) (181.2036, -14.3748) (184.8216, -14.3359) (188.3219, -14.2957) (191.7011, -14.2566) (194.9552, -14.2171) (198.0817, -14.1783) (201.0766, -14.1393) (203.9375, -14.1021) (206.6609, -14.0643) (209.2442, -14.0284) (211.6849, -13.9935) (213.9802, -13.959) (216.1277, -13.9267) (218.1257, -13.8961) (219.9714, -13.8664) (221.663, -13.8394) (223.1992, -13.8136) (224.5774, -13.7911) (225.7973, -13.77) (226.8565, -13.7518) (227.7552, -13.7365) (228.4879, -13.723) (229.184, -13.7115) (229.5963, -13.7034) (229.8419, -13.6991) (229.8922, -13.6984) knots 0 0 0 0 0 0.003306 0.005253 0.00752 0.010062 0.01285 0.015861 0.019079 0.022488 0.026078 0.029837 0.033757 0.037828 0.042045 0.046398 0.050884 0.055494 0.060224 0.065069 0.070023 0.075082 0.080241 0.085495 0.090841 0.096274 0.101791 0.107386 0.113057 0.118799 0.124609 0.130484 0.136419 0.142412 0.148458 0.154554 0.160697 0.166884 0.17311 0.179374 0.185671 0.191998 0.198352 0.20473 0.211128 0.217543 0.223972 0.230412 0.23686 0.243312 0.249765 0.256217 0.262663 0.2691 0.275526 0.281941 0.288345 0.294734 0.301105 0.307451 0.313767 0.320049 0.326294 0.332498 0.338659 0.344773 0.350837 0.356848 0.362801 0.368695 0.374525 0.380288 0.38598 0.391599 0.39714 0.4026 0.407976 0.413263 0.418458 0.423557 0.428556 0.433452 0.438241 0.442917 0.447478 0.451919 0.456236 0.460425 0.464482 0.468403 0.472185 0.475825 0.479322 0.482675 0.485889 0.48897 0.49193 0.494788 0.497572 0.50031 0.503032 0.505769 0.508552 0.511409 0.514365 0.517441 0.520647 0.523991 0.527474 0.531098 0.534861 0.538758 0.542789 0.546947 0.551231 0.555634 0.560154 0.564786 0.569527 0.574371 0.579315 0.584356 0.58949 0.594712 0.60002 0.605409 0.610877 0.61642 0.622034 0.627716 0.633463 0.639271 0.645138 0.651061 0.657035 0.663059 0.669128 0.675241 0.681393 0.687582 0.693804 0.700057 0.706341 0.712655 0.718998 0.725365 0.731751 0.738149 0.744556 0.750969 0.757385 0.7638 0.770211 0.776616 0.783011 0.789393 0.795759 0.802106 0.808429 0.814727 0.820996 0.827232 0.833433 0.839595 0.845714 0.851788 0.857813 0.863785 0.869702 0.875558 0.881352 0.887078 0.892735 0.898316 0.90382 0.909242 0.914577 0.919822 0.924972 0.930023 0.93497 0.939808 0.944533 0.949139 0.95362 0.95797 0.962183 0.966252 0.970169 0.973927 0.977515 0.980924 0.984141 0.987151 0.989939 0.99248 0.994747 0.996694 1 1 1 1 1
  circle A0 centre (0, 0) radius 5.15
  line L0 (-29.05, 5.1) -> (-39.25, 5.1)
  line L1 (-39.25, 5.1) -> (-39.25, 0.9)
  line L2 (-39.25, 0.9) -> (-29.05, 0.9)
  line L3 (-29.05, 0.9) -> (-29.05, 5.1)
  line L4 (-29.05, 5.1) -> (-39.25, 0.9) construction
  line L5 (-39.25, 5.1) -> (-29.05, 0.9) construction
  line L6 (-70.9, 3.9) -> (-60.7, 3.9)
  line L7 (-60.7, 3.9) -> (-60.7, 8.1)
  line L8 (-60.7, 8.1) -> (-70.9, 8.1)
  line L9 (-70.9, 8.1) -> (-70.9, 3.9)
  line L10 (-70.9, 3.9) -> (-60.7, 8.1) construction
  line L11 (-60.7, 3.9) -> (-70.9, 8.1) construction
  line L12 (54.9, 4.1) -> (65.1, 4.1)
  line L13 (65.1, 4.1) -> (65.1, -0.1)
  line L14 (65.1, -0.1) -> (54.9, -0.1)
  line L15 (54.9, -0.1) -> (54.9, 4.1)
  line L16 (54.9, 4.1) -> (65.1, -0.1) construction
  line L17 (65.1, 4.1) -> (54.9, -0.1) construction
  line L18 (109.9, -1.9) -> (120.1, -1.9)
  line L19 (120.1, -1.9) -> (120.1, -6.1)
  line L20 (120.1, -6.1) -> (109.9, -6.1)
  line L21 (109.9, -6.1) -> (109.9, -1.9)
  line L22 (109.9, -1.9) -> (120.1, -6.1) construction
  line L23 (120.1, -1.9) -> (109.9, -6.1) construction
  point P0 (229.5755, -13.6106)
  point P1 (229.1796, -13.5013)
  point P2 (228.6261, -13.3487)
  point P3 (227.9153, -13.1528)
  point P4 (227.0478, -12.9149)
  point P5 (226.0244, -12.6347)
  point P6 (224.8458, -12.3137)
  point P7 (223.5134, -11.9522)
  point P8 (222.0284, -11.5516)
  point P9 (220.3919, -11.1123)
  point P10 (218.6056, -10.6357)
  point P11 (216.6708, -10.123)
  point P12 (214.5898, -9.5751)
  point P13 (212.3638, -8.9939)
  point P14 (209.9954, -8.3805)
  point P15 (207.4868, -7.7363)
  point P16 (204.8398, -7.0625)
  point P17 (202.0571, -6.3611)
  point P18 (199.1415, -5.6336)
  point P19 (196.0954, -4.8816)
  point P20 (192.9216, -4.1065)
  point P21 (189.6234, -3.3101)
  point P22 (186.2035, -2.4943)
  point P23 (182.6657, -1.6609)
  point P24 (179.0124, -0.8111)
  point P25 (175.248, 0.0529)
  point P26 (171.3752, 0.9297)
  point P27 (167.3986, 1.8169)
  point P28 (163.321, 2.7134)
  point P29 (159.147, 3.617)
  point P30 (154.8803, 4.5261)
  point P31 (150.5252, 5.4389)
  point P32 (146.0855, 6.3537)
  point P33 (141.5661, 7.2686)
  point P34 (136.9704, 8.1819)
  point P35 (132.3036, 9.0917)
  point P36 (127.5703, 9.9964)
  point P37 (122.7747, 10.8942)
  point P38 (117.9215, 11.7832)
  point P39 (113.0152, 12.6619)
  point P40 (108.0612, 13.5285)
  point P41 (103.0641, 14.3813)
  point P42 (98.0285, 15.2183)
  point P43 (92.9599, 16.0381)
  point P44 (87.8625, 16.8391)
  point P45 (82.7421, 17.6192)
  point P46 (77.6032, 18.3772)
  point P47 (72.4514, 19.1113)
  point P48 (67.2912, 19.8203)
  point P49 (62.1283, 20.502)
  point P50 (56.9674, 21.1549)
  point P51 (51.8139, 21.7784)
  point P52 (46.6728, 22.3701)
  point P53 (41.5494, 22.9292)
  point P54 (36.4487, 23.4539)
  point P55 (31.3516, 23.9432)
  point P56 (26.2698, 24.3871)
  point P57 (21.2254, 24.7829)
  point P58 (16.2232, 25.1297)
  point P59 (11.2688, 25.4269)
  point P60 (6.3675, 25.6745)
  point P61 (1.5244, 25.8714)
  point P62 (-3.2556, 26.0185)
  point P63 (-7.9669, 26.1147)
  point P64 (-12.605, 26.1607)
  point P65 (-17.1647, 26.1565)
  point P66 (-21.6414, 26.1029)
  point P67 (-26.03, 25.9999)
  point P68 (-30.3262, 25.8485)
  point P69 (-34.5251, 25.6495)
  point P70 (-38.6223, 25.4038)
  point P71 (-42.6138, 25.1124)
  point P72 (-46.4949, 24.7767)
  point P73 (-50.2615, 24.398)
  point P74 (-53.9103, 23.9777)
  point P75 (-57.4369, 23.5172)
  point P76 (-60.838, 23.0185)
  point P77 (-64.1097, 22.4827)
  point P78 (-67.2491, 21.9117)
  point P79 (-70.2526, 21.3079)
  point P80 (-73.1173, 20.6725)
  point P81 (-75.8404, 20.0075)
  point P82 (-78.4195, 19.3151)
  point P83 (-80.8514, 18.5968)
  point P84 (-83.1341, 17.8549)
  point P85 (-85.2656, 17.091)
  point P86 (-87.2437, 16.3068)
  point P87 (-89.0663, 15.5041)
  point P88 (-90.7324, 14.6848)
  point P89 (-92.2399, 13.8505)
  point P90 (-93.5876, 13.0024)
  point P91 (-94.775, 12.1424)
  point P92 (-95.8001, 11.2711)
  point P93 (-96.6631, 10.3901)
  point P94 (-97.363, 9.5007)
  point P95 (-97.8994, 8.6033)
  point P96 (-98.2716, 7.6987)
  point P97 (-98.4805, 6.7876)
  point P98 (-98.5252, 5.8707)
  point P99 (-98.4071, 4.9603)
  point P100 (-98.1267, 4.0689)
  point P101 (-97.6849, 3.1969)
  point P102 (-97.0825, 2.3442)
  point P103 (-96.32, 1.5114)
  point P104 (-95.3988, 0.6992)
  point P105 (-94.3198, -0.0929)
  point P106 (-93.0847, -0.8642)
  point P107 (-91.6947, -1.6144)
  point P108 (-90.1515, -2.3431)
  point P109 (-88.4571, -3.0499)
  point P110 (-86.613, -3.7345)
  point P111 (-84.6215, -4.3967)
  point P112 (-82.4847, -5.0362)
  point P113 (-80.2051, -5.6525)
  point P114 (-77.7848, -6.246)
  point P115 (-75.2265, -6.8157)
  point P116 (-72.5328, -7.3621)
  point P117 (-69.7064, -7.8852)
  point P118 (-66.7502, -8.3843)
  point P119 (-63.6672, -8.8597)
  point P120 (-60.4603, -9.3121)
  point P121 (-57.133, -9.7408)
  point P122 (-53.6883, -10.1467)
  point P123 (-50.1292, -10.5299)
  point P124 (-46.4597, -10.8909)
  point P125 (-42.6832, -11.2303)
  point P126 (-38.8031, -11.5482)
  point P127 (-34.823, -11.846)
  point P128 (-30.7468, -12.1235)
  point P129 (-26.5785, -12.3824)
  point P130 (-22.3217, -12.6229)
  point P131 (-17.9803, -12.8463)
  point P132 (-13.5587, -13.0537)
  point P133 (-9.0605, -13.2456)
  point P134 (-4.4905, -13.4237)
  point P135 (0.1474, -13.5886)
  point P136 (4.849, -13.7415)
  point P137 (9.6099, -13.8842)
  point P138 (14.4255, -14.0175)
  point P139 (19.2912, -14.1423)
  point P140 (24.2029, -14.2603)
  point P141 (29.1558, -14.3722)
  point P142 (34.1617, -14.4796)
  point P143 (39.2237, -14.5759)
  point P144 (44.3121, -14.6593)
  point P145 (49.423, -14.7298)
  point P146 (54.5505, -14.7888)
  point P147 (59.6901, -14.8374)
  point P148 (64.8368, -14.8761)
  point P149 (69.9851, -14.9057)
  point P150 (75.1303, -14.9272)
  point P151 (80.2674, -14.9409)
  point P152 (85.3913, -14.9483)
  point P153 (90.4968, -14.9493)
  point P154 (95.5789, -14.9453)
  point P155 (100.6326, -14.9363)
  point P156 (105.6533, -14.9226)
  point P157 (110.6353, -14.9057)
  point P158 (115.574, -14.8853)
  point P159 (120.4648, -14.8616)
  point P160 (125.3027, -14.8358)
  point P161 (130.0823, -14.8075)
  point P162 (134.7998, -14.7774)
  point P163 (139.4498, -14.7457)
  point P164 (144.0277, -14.7123)
  point P165 (148.5293, -14.6776)
  point P166 (152.9501, -14.6421)
  point P167 (157.285, -14.6058)
  point P168 (161.5303, -14.5684)
  point P169 (165.6817, -14.5303)
  point P170 (169.7345, -14.492)
  point P171 (173.6849, -14.4529)
  point P172 (177.5292, -14.4136)
  point P173 (181.2631, -14.3741)
  point P174 (184.883, -14.3347)
  point P175 (188.3852, -14.2949)
  point P176 (191.7661, -14.2554)
  point P177 (195.0221, -14.2161)
  point P178 (198.1502, -14.177)
  point P179 (201.1468, -14.1384)
  point P180 (204.0092, -14.1007)
  point P181 (206.7341, -14.0633)
  point P182 (209.3188, -14.0271)
  point P183 (211.7608, -13.992)
  point P184 (214.0574, -13.9578)
  point P185 (216.2063, -13.9254)
  point P186 (218.2054, -13.8945)
  point P187 (220.0521, -13.8651)
  point P188 (221.7449, -13.8378)
  point P189 (223.2819, -13.8124)
  point P190 (224.6613, -13.7894)
  point P191 (225.882, -13.7686)
  point P192 (226.9427, -13.7504)
  point P193 (227.8417, -13.7347)
  point P194 (228.5791, -13.7216)
  point P195 (229.1532, -13.7117)
  point P196 (229.5636, -13.7042)
  point P197 (229.8101, -13.6997)
  point P198 (-34.15, 3)
  point P199 (-65.8, 6)
  dimension "d8" = 10.3
  dimension "d9" = 98.7
  dimension "d63" = 10.2
  dimension "d64" = 4.2
  dimension "d66" = 10.2
  dimension "d67" = 4.2
  dimension "d138" = 34.15
  dimension "d139" = 3
  dimension "d140" = 65.8
  dimension "d141" = 6
  dimension "d219" = 10.2
  dimension "d220" = 4.2
  dimension "d221" = 60
  dimension "d222" = 2
  dimension "d223" = 10.2
  dimension "d224" = 4.2
  dimension "d225" = 115
  dimension "d226" = 4
  constraints: 48 end point, 8 midpoint, 8 parallel, 4 horizontal, 4 perpendicular, 1 centre point, 201 other
  measures "d8" diameter of A0
  measures "d9" distance of A0.centre point (-98.525, 5.871)
  measures "d63" distance of L2.end L1.end
  measures "d64" distance of L1.end L0.end
  measures "d66" distance of L8.end L7.end
  measures "d67" distance of L7.end L6.end
  measures "d138" horizontal distance of point (0, 0) point (-34.15, 3)
  measures "d139" vertical distance of point (0, 0) point (-34.15, 3)
  measures "d140" horizontal distance of point (0, 0) point (-65.8, 6)
  measures "d141" vertical distance of point (0, 0) point (-65.8, 6)
  measures "d219" distance of L13.end L14.end
  measures "d220" distance of L12.end L13.end
  measures "d221" horizontal distance of point (60, 2) point (0, 0)
  measures "d222" vertical distance of point (60, 2) point (0, 0)
  measures "d223" distance of L19.end L20.end
  measures "d224" distance of L18.end L19.end
  measures "d225" horizontal distance of point (115, -4) point (0, 0)
  measures "d226" vertical distance of point (115, -4) point (0, 0)